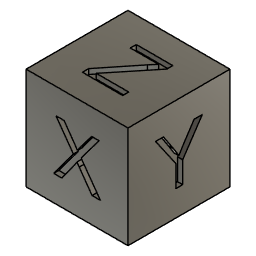
Cubo_XYZ (Autodesk Fusion 360 design; units mm, degrees)
Autodesk Fusion 360 part; units mm, degrees
sketch "Esboço1" plane through (0, 0, 0) normal (0, 0, 1) x (1, 0, 0)
  line L0 (0, 0) -> (20, 0)
  line L1 (20, 0) -> (20, 20)
  line L2 (20, 20) -> (0, 20)
  line L3 (0, 20) -> (0, 0)
  dimension "d1" = 20
  dimension "d2" = 20
  constraint horizontal L0
  constraint vertical L1
  constraint horizontal L2
  constraint vertical L3
  constraint coincident L0.start L3.end
  measures "d1" distance of L0.start L0.end
  measures "d2" distance of L0.start L2.end
extrude "Extrusão1" add sketch "Esboço1" along normal blind 20
sketch "Esboço2" plane through (20, 0, 0) normal (1, 0, 0) x (0, 1, 0)
  line L0 (0, 0) -> (20, 0)
  line L1 (20, 0) -> (20, 20)
  line L2 (20, 20) -> (0, 20)
  line L3 (0, 20) -> (0, 0)
  line L4 (20, 0) -> (0, 0) construction
  line L5 (0, 0) -> (0, 20) construction
  line L6 (0, 20) -> (20, 20) construction
  line L7 (20, 20) -> (20, 0) construction
  dimension "d5" = 10
  text T0 "Y" font "Arial" height 10 align centre middle in box 20 x 20 at (20, 0) x (-1, 0) y (0, 1) spacing 1
  constraint coincident L0.start
  constraint coincident L1.end
sketch "Esboço3" plane through (0, 0, 0) normal (0, -1, 0) x (1, 0, 0)
  line L0 (0, 0) -> (20, 0)
  line L1 (20, 0) -> (20, 20)
  line L2 (20, 20) -> (0, 20)
  line L3 (0, 20) -> (0, 0)
  line L4 (0, 0) -> (20, 0) construction
  line L5 (20, 0) -> (20, 20) construction
  line L6 (20, 20) -> (0, 20) construction
  line L7 (0, 20) -> (0, 0) construction
  dimension "d6" = 10
  text T0 "X" font "Arial" height 10 align centre middle in box 20 x 20 at (0, 0) x (1, 0) y (0, 1) spacing 1
  constraint coincident L0.end
  constraint coincident L2.end
sketch "Esboço4" plane through (0, 0, 20) normal (0, 0, 1) x (-1, 0, 0)
  line L0 (0, -20) -> (0, 0)
  line L1 (0, 0) -> (-20, 0)
  line L2 (-20, 0) -> (-20, -20)
  line L3 (-20, -20) -> (0, -20)
  line L4 (0, 0) -> (-20, 0) construction
  line L5 (-20, 0) -> (-20, -20) construction
  line L6 (-20, -20) -> (0, -20) construction
  line L7 (0, -20) -> (0, 0) construction
  dimension "d7" = 10
  text T0 "Z" font "Arial" height 10 align centre middle in box 20 x 20 at (0, 0) x (-1, 0) y (0, -1) spacing 1
  constraint coincident L1.end
  constraint coincident L0.start
extrude "Extrusão2" cut sketch "Esboço4" against normal blind 1 text T0
extrude "Extrusão3" cut sketch "Esboço2" against normal blind 1 text T0
extrude "Extrusão4" cut sketch "Esboço3" against normal blind 1 text T0
sketch "Esboço5" plane through (0, 0, 0) normal (-1, 0, 0) x (0, -1, 0)
  line L0 (-20, 0) -> (0, 0)
  line L1 (0, 0) -> (0, 20)
  line L2 (0, 20) -> (-20, 20)
  line L3 (-20, 20) -> (-20, 0)
  line L4 (-24.1421, 10) -> (-10, -4.1421) construction
  line L5 (-10, -4.1421) -> (4.1421, 10) construction
  line L6 (4.1421, 10) -> (-10, 24.1421) construction
  line L7 (-10, 24.1421) -> (-24.1421, 10) construction
  dimension "d14" = 7
  text T0 "2x2" font "Arial" height 7 bold align centre middle in box 20 x 20 at (-24.1421, 10) x (0.707107, -0.707107) y (0.707107, 0.707107) spacing 1
extrude "Extrusão5" cut sketch "Esboço5" against normal blind 1 text T0
named bodies: "Cube_2x2"
